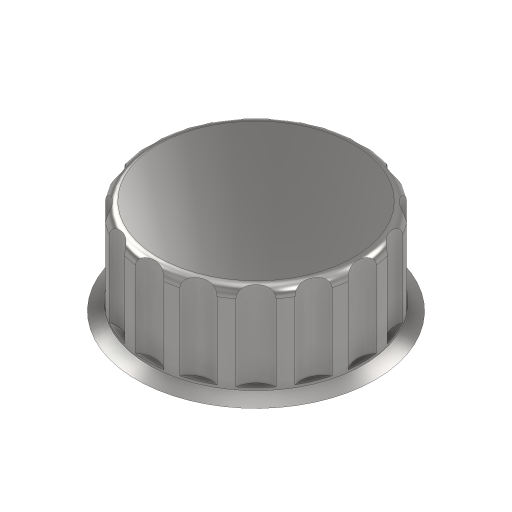
# Autodesk Inventor part: Part008Handwheel
Saved by Autodesk Inventor 2023.2 (Build 272271030, 271C)
## iProperties
Created: 2023-09-07
Part Number: Part008Handwheel
Material: Stainless Steel
Document SubType Name: Modeling
Designer: User
Density: 8 g/cm^3
Appearance: Semi-Polished
Author: User
Autodesk Inventor part; units mm, degrees
ref_plane "YZ Plane" through (0, 0, 0) normal (1, 0, 0) x (0, 1, 0)
ref_plane "XZ Plane" through (0, 0, 0) normal (0, 1, 0) x (-1, 0, 0)
sketch "Sketch1" plane through (0, 0, 0) normal (0, 0, 1) x (1, 0, 0)
  line L0 (0, 18) -> (-4, 18)
  line L1 (-4, 18) -> (-4, 0)
  line L2 (-4, 0) -> (-6, 0)
  line L3 (-6, 0) -> (-6, 18)
  line L4 (-6, 18) -> (-20.5, 18)
  line L5 (-20.5, 18) -> (-20.5, 0)
  line L6 (-20.5, 0) -> (-25, 0)
  line L7 (-25, 0) -> (-22.5, 1.4434)
  line L8 (-22.5, 1.4434) -> (-22.5, 18)
  arc A0 (-20.5, 20) -> (-22.5, 18) centre (-20.5, 18) ccw
  line L9 (-20.5, 20) -> (0, 20)
  line L10 (0, 20) -> (0, 18)
  line L11 (0, -4.0828) -> (0, 24.4971) projected
  point P0 (0, 0)
  point P1 (-5, 0)
  dimension "d0" = 20
  dimension "d1" = 2
  dimension "d2" = 2
  dimension "d3" = 12
  dimension "d4" = 8
  dimension "d5" = 50
  dimension "d7" = 30
  dimension "d8" = 41
  constraints: 22 end point, 7 point on line, 4 perpendicular, 2 horizontal, 2 point on circle, 1 centre point, 1 coincident, 1 midpoint, 1 parallel, 1 tangent, 1 vertical
  measures "d0" distance from line of point (-5, 0) L9
  measures "d1" distance between parallel lines of L4 L9
  measures "d2" radius of A0
  measures "d3" diameter of L3 L11
  measures "d4" diameter of L1 L11
  measures "d5" diameter of L6.end L11
  measures "d7" angle of L7 L6
  measures "d8" diameter of L5 L11
revolve "Revolution1" add sketch "Sketch1" angle 360 about axis through (0, -10, 0) along (0, 1, 0)
ref_plane "Work Plane1" through (0, 2, 0) normal (0, -1, 0) x (1, 0, 0)
sketch "Sketch2" plane through (0, 2, 0) normal (0, -1, 0) x (1, 0, 0)
  circle A0 centre (26, 0) radius 4.75
  point P0 (0, 0)
  dimension "d13" = 4.75
  dimension "d14" = 26
  constraints: 1 centre point, 1 horizontal alignment
  measures "d13" radius of A0
  measures "d14" distance of A0.centre point (0, 0)
extrude "Extrusion1" cut sketch "Sketch2" against normal through all
pattern_circular "Circular Pattern1" count 16 over 360 about axis through (0, 0.7217, 0) along (0, 1, 0) of "Extrusion1"
sketch "Sketch4" plane through (0, 0, 0) normal (0, -1, 0) x (1, 0, 0)
  circle A0 centre (0, 0) radius 4 projected
  line L0 (-1, -0.7778) -> (1, -0.7778)
  line L1 (1, -0.7778) -> (1, -5)
  line L2 (1, -5) -> (-1, -5)
  line L3 (-1, -5) -> (-1, -0.7778)
  point P0 (0, -0.7778)
  dimension "d20" = 2
  dimension "d22" = 9
  constraints: 8 end point, 2 parallel, 1 horizontal, 1 midpoint, 1 perpendicular, 1 vertical alignment
  measures "d20" distance between parallel lines of L1 L3
extrude "Extrusion2" cut sketch "Sketch4" against normal up to surface (18 mm away) contours L3 L0 L1 A0 | A0 L1 L2 L3 picked at (-0.1122, -1.8471)
body "Solid1"
